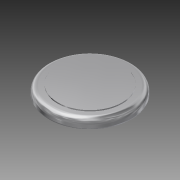
# Autodesk Inventor part: cr1620
Saved by Autodesk Inventor 2014 (Build 180170000, 170)
## iProperties
Created: 2014-11-29
Part Number: cr1620
Material: Aluminum 6061
Document SubType Name: Modeling
Designer: DV
Mass: 1.02527 g
Surface Area: 4.76453 cm^2
Volume: 0.37833 cm^3
Density: 2.71 g/cm^3
Appearance: Aluminum - Flat
Author: DV
Autodesk Inventor part; units mm, degrees
ref_plane "YZ Plane" through (0, 0, 0) normal (1, 0, 0) x (0, 1, 0)
ref_plane "XZ Plane" through (0, 0, 0) normal (0, 1, 0) x (-1, 0, 0)
ref_plane "XY Plane" through (0, 0, 0) normal (0, 0, 1) x (1, 0, 0)
sketch "Sketch1" plane through (0, 0, 0) normal (0, 0, 1) x (1, 0, 0)
  line L0 (0, 0) -> (7.619, 0)
  line L1 (8, 0.381) -> (8, 0.8508)
  line L2 (8, 2) -> (0, 2)
  line L3 (0, 2) -> (0, 0)
  arc A0 (7.619, 0) -> (8, 0.381) centre (7.619, 0.381) ccw
  arc A1 (8, 0.8508) -> (6.984, 1.8668) centre (6.984, 0.8508) ccw
  line L4 (6.119, 2) -> (6.119, 1.7889)
  line L5 (6.119, 1.7889) -> (6.2213, 1.7889)
  line L6 (6.2213, 1.7889) -> (6.2213, 1.8668)
  line L7 (6.2213, 1.8668) -> (6.984, 1.8668)
  line L8 (6.119, 2) -> (0, 2)
  point P0 (8, 0)
  dimension "d1" = 2
  dimension "d2" = 0.381
  dimension "d3" = 1.016
  constraints: 18 end point, 4 perpendicular, 4 point on circle, 4 point on line, 4 tangent, 3 parallel, 2 centre point, 1 collinear, 1 horizontal
  measures "d1" distance of L2.start point (8, 0)
  measures "d2" radius of A0
  measures "d3" radius of A1
revolve "Revolution1" add sketch "Sketch1" angle 360 about axis through (0, 2, 0) along (0, -1, 0)
body "Solid1"
